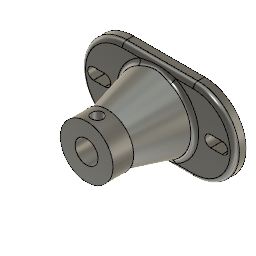
_casting.41a3ebeb-be81-4f54-89be-00689bddbda9 (Autodesk Fusion 360 design; units mm, degrees)
Autodesk Fusion 360 part; units mm, degrees
sketch "Sketch1" plane through (0, 0, 0) normal (0, 1, 0) x (1, 0, 0)
  arc A0 (97.9117, -72) -> (97.9117, 0) centre (97.9999, -36) ccw
  arc A1 (36, 0) -> (36, -72) centre (36, -36) ccw
  line L0 (36, -72) -> (97.9117, -72)
  line L1 (36, 0) -> (97.9117, 0)
  line L2 (66.9558, 0) -> (66.9558, -72)
  line L3 (122.9558, -41) -> (112.9558, -41)
  line L4 (112.9558, -41) -> (112.9558, -31)
  line L5 (112.9558, -31) -> (122.9558, -31)
  line L6 (122.9558, -31) -> (122.9558, -41)
  line L7 (122.9558, -41) -> (112.9558, -31) construction
  line L8 (112.9558, -41) -> (122.9558, -31) construction
  arc A2 (122.9558, -41) -> (122.9558, -31) centre (122.9558, -36) ccw
  arc A3 (112.9558, -31) -> (112.9558, -41) centre (112.9558, -36) ccw
  line L9 (66.9558, -36) -> (15.9558, -36)
  line L10 (20.9558, -41) -> (10.9558, -41)
  line L11 (10.9558, -41) -> (10.9558, -31)
  line L12 (10.9558, -31) -> (20.9558, -31)
  line L13 (20.9558, -31) -> (20.9558, -41)
  line L14 (20.9558, -41) -> (10.9558, -31) construction
  line L15 (10.9558, -41) -> (20.9558, -31) construction
  arc A4 (20.9558, -41) -> (20.9558, -31) centre (20.9558, -36) ccw
  arc A5 (10.9558, -31) -> (10.9558, -41) centre (10.9558, -36) ccw
  point P0 (117.9558, -36)
  point P1 (15.9558, -36)
  dimension "d10" = 51
  dimension "d11" = 10
  dimension "d12" = 10
  constraint midpoint L1 L2.start
  constraint midpoint L0 L2.end
  constraint perpendicular L0 L2
  constraint perpendicular L3 L4
  constraint parallel L3 L5
  constraint parallel L4 L6
  constraint horizontal L3
  constraint coincident L7 P0
  constraint coincident L8 P0
  constraint midpoint L6 A2.centre
  constraint midpoint L4 A3.centre
  constraint midpoint L2 L9.start
  constraint perpendicular L2 L9
  constraint perpendicular L10 L11
  constraint parallel L10 L12
  constraint parallel L11 L13
  constraint horizontal L10
  constraint coincident L14 P1
  constraint coincident L15 P1
  constraint coincident P1 L9.end
  constraint midpoint L13 A4.centre
  constraint midpoint L11 A5.centre
  measures "d10" distance of L9.start P1
  measures "d11" distance of L10.end L11.end
  measures "d12" distance of L11.end L12.end
extrude "Extrude1" add sketch "Sketch1" along normal blind 10
ref_plane "WorkPlane1" through (0, 0, 36) normal (0, 0, 1) x (1, 0, 0)
sketch "Sketch2" plane through (0, 0, 36) normal (0, 0, 1) x (1, 0, 0)
sketch "Sketch3" plane through (0, 0, 0) normal (0, -1, 0) x (1, 0, 0)
  arc A0 (122.9558, 31) -> (122.9558, 41) centre (122.9558, 36) ccw
  line L0 (122.9558, 31) -> (112.9558, 31)
  arc A1 (112.9558, 41) -> (112.9558, 31) centre (112.9558, 36) ccw
  line L1 (112.9558, 41) -> (122.9558, 41)
  arc A2 (20.9558, 31) -> (20.9558, 41) centre (20.9558, 36) ccw
  line L2 (20.9558, 31) -> (10.9558, 31)
  arc A3 (10.9558, 41) -> (10.9558, 31) centre (10.9558, 36) ccw
  line L3 (10.9558, 41) -> (20.9558, 41)
  line L4 (97.9117, 72) -> (36, 72)
  arc A4 (36, 72) -> (36, 0) centre (36, 36) ccw
  line L5 (36, 0) -> (97.9117, 0)
  arc A5 (97.9117, 0) -> (97.9117, 72) centre (97.9999, 36) ccw
  line L6 (66.9558, 0) -> (66.9558, 72)
  line L7 (0, 36) -> (0.0524, 37.9413)
  line L8 (66.9558, 0) -> (66.9558, 36)
  circle A6 centre (66.9558, 36) radius 32.5
  dimension "d16" = 36
  dimension "d17" = 65
  constraint midpoint L5 L6.start
  constraint midpoint L4 L6.end
  constraint midpoint A4 L7.start
  constraint coincident A4 L7.end
  constraint perpendicular L5 L8
  constraint coincident L8.end A6.centre
  measures "d16" distance of L6.start L8.end
  measures "d17" diameter of A6
ref_plane "WorkPlane2" through (0, -44, 0) normal (0, 1, 0) x (0, 0, 1)
sketch "Sketch4" plane through (0, -44, 0) normal (0, 1, 0) x (1, 0, 0)
  circle A0 centre (66.9558, -36) radius 21
  point P0 (66.9558, -36)
  dimension "d19" = 42
  constraint coincident P0 A0.centre
  measures "d19" diameter of A0
loft "Loft1" add profiles "Sketch3", "Sketch4" section 1 contours L6 L8 A6 | L6 L8 A6 section 2
sketch "Sketch5" plane through (0, -44, 0) normal (0, -1, 0) x (1, 0, 0)
  circle A0 centre (66.9558, 36) radius 21
  circle A1 centre (66.9558, 36) radius 23
  dimension "d20" = 46
  constraint concentric A0 A1
  measures "d20" diameter of A1
extrude "Extrude2" add sketch "Sketch5" along normal blind 18 contours A0 | A1
ref_plane "WorkPlane3" through (0, 0, 36) normal (0, 0, 1) x (1, 0, 0)
sketch "Sketch6" plane through (0, 0, 36) normal (0, 0, 1) x (1, 0, 0)
  line L0 (97.9117, 10) -> (36, 10)
  line L1 (66.9558, 10) -> (66.9558, -40)
  line L2 (66.9558, 10) -> (36.9558, 10)
  line L3 (36.9558, 10) -> (50, -40)
  line L4 (50, -40) -> (66.9558, -40)
  dimension "d24" = 50
  dimension "d25" = 30
  constraint midpoint L0 L1.start
  constraint perpendicular L0 L1
  constraint perpendicular L1 L2
  constraint perpendicular L1 L4
  measures "d24" distance of L1.start L1.end
  measures "d25" distance of L1.start L2.end
revolve "Revolve1" cut sketch "Sketch6" angle 360 about axis through (66.9558, 10, 36) along (0, -1, 0)
fillet "Fillet1" radius 4 1 edges at (51.1474, -40, 42.1315)
sketch "Sketch7" plane through (0, -62, 0) normal (0, -1, 0) x (1, 0, 0)
  circle A0 centre (66.9558, 36) radius 23
  circle A1 centre (66.9558, 36) radius 10
  dimension "d28" = 20
  constraint concentric A0 A1
  measures "d28" diameter of A1
extrude "Extrude3" cut sketch "Sketch7" against normal blind 22 contours A1
ref_plane "WorkPlane4" through (0, 0, 36) normal (0, 0, 1) x (1, 0, 0)
sketch "Sketch8" plane through (0, 0, 36) normal (0, 0, 1) x (1, 0, 0)
  line L0 (43.9558, -44) -> (89.9558, -44)
  line L1 (76.9558, -62) -> (56.9558, -62)
  line L2 (66.9558, -44) -> (66.9558, -62)
  line L3 (66.9558, -44) -> (66.9558, -53)
  circle A0 centre (66.9558, -53) radius 5
  dimension "d32" = 9
  dimension "d33" = 10
  constraint midpoint L0 L2.start
  constraint midpoint L1 L2.end
  constraint perpendicular L0 L3
  constraint coincident L3.end A0.centre
  measures "d32" distance of L2.start L3.end
  measures "d33" diameter of A0
extrude "Extrude4" cut sketch "Sketch8" along normal blind 40
fillet "Fillet2" radius 4 5 edges at (66.9558, 0, 0) (0, 0, 36) (66.9558, 0, 72) (36.6552, 0, 47.7525) (134, 0, 36)
